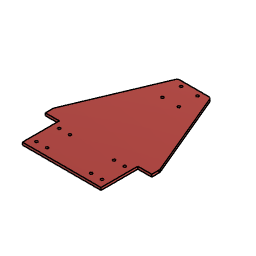
Chassis v45 (Autodesk Fusion 360 design; units mm, degrees)
Autodesk Fusion 360 part; units mm, degrees
sketch "Main" plane through (0, 0, 0) normal (0, 0, 1) x (1, 0, 0)
  line L0 (0, 55) -> (45, 162)
  line L1 (45, 162) -> (85, 162)
  line L2 (85, 162) -> (130, 55)
  line L3 (113, 0) -> (17, 0)
  line L4 (65, 0) -> (65, 162) construction
  line L5 (0, 55) -> (0, 45)
  line L6 (0, 45) -> (17, 45)
  line L7 (17, 45) -> (17, 0)
  line L8 (130, 55) -> (130, 45)
  line L9 (130, 45) -> (113, 45)
  line L10 (113, 45) -> (113, 0)
  dimension "d2" = 162
  dimension "d6" = 55
  dimension "d9" = 40
  dimension "d45" = 130
  dimension "d47" = 17
  dimension "d48" = 17
  dimension "d49" = 10
  dimension "d50" = 10
  constraint horizontal L0.start L2.end
  constraint midpoint L3 L4.start
  constraint perpendicular L3 L4
  constraint midpoint L1 L4.end
  constraint vertical L5
  constraint perpendicular L5 L6
  constraint coincident L3 L7.end
  constraint perpendicular L3 L7
  constraint vertical L8
  constraint perpendicular L8 L9
  constraint coincident L3 L10.end
  constraint perpendicular L3 L10
  constraint horizontal L3
  constraint coincident L3.start L10.end
  constraint vertical origin L5.end
  constraint coincident L3.end L7.end
  constraint horizontal origin L3.end
  measures "d2" distance of L1 L3
  measures "d6" distance of origin L0.start
  measures "d9" distance of L0.end L1.end
  measures "d45" distance of L5 L8
  measures "d47" distance of L5.end L6.end
  measures "d48" distance of L8.end L9.end
  measures "d49" distance of L2.end L8.end
  measures "d50" distance of L0.start L5.end
extrude "Extrude1" add sketch "Main" along normal blind 3
sketch "Head Tube Holes" plane through (0, 0, 3) normal (0, 0, 1) x (-1, 0, 0)
  line L0 (-17, 0) -> (-113, 0)
  line L1 (-130, -55) -> (-85, -162)
  line L2 (-85, -162) -> (-45, -162)
  line L3 (-45, -162) -> (0, -55)
  circle A0 centre (-55, -156) radius 1.55
  line L4 (-65, -162) -> (-65, 0) construction
  circle A1 centre (-75, -156) radius 1.55
  circle A2 centre (-55, -133) radius 1.55
  circle A3 centre (-75, -133) radius 1.55
  line L5 (0, -55) -> (0, -45)
  line L6 (0, -45) -> (-17, -45)
  line L7 (-17, -45) -> (-17, 0)
  line L8 (-113, 0) -> (-113, -45)
  line L9 (-113, -45) -> (-130, -45)
  line L10 (-130, -45) -> (-130, -55)
  dimension "d19" = 3.1
  dimension "d20" = 6
  dimension "d21" = 10
  dimension "d24" = -20
  dimension "d25" = 23
  constraint midpoint L2 L4.start
  constraint midpoint L0 L4.end
  measures "d19" diameter of A0
  measures "d20" distance of L2 A0.centre
  measures "d21" distance of A0.centre L4
extrude "Extrude2" cut sketch "Head Tube Holes" against normal up to surface (3 mm away) contours A0 | A1 | A2 | A3
sketch "Motor Box Holes" plane through (0, 0, 3) normal (0, 0, 1) x (-1, 0, 0)
  circle A0 centre (-75, -156) radius 1.55
  circle A1 centre (-55, -156) radius 1.55
  circle A2 centre (-75, -133) radius 1.55
  circle A3 centre (-55, -133) radius 1.55
  line L0 (-17, 0) -> (-113, 0)
  line L1 (-17, -37) -> (-113, -37) construction
  circle A4 centre (-25, -37) radius 1.55
  circle A5 centre (-38.1, -37) radius 1.55
  circle A6 centre (-25, -9.1) radius 1.55
  circle A7 centre (-38.1, -9.1) radius 1.55
  circle A8 centre (-105, -37) radius 1.55
  circle A9 centre (-91.9, -37) radius 1.55
  circle A10 centre (-105, -9.1) radius 1.55
  circle A11 centre (-91.9, -9.1) radius 1.55
  line L2 (-17, -45) -> (-17, 0)
  line L3 (-113, 0) -> (-113, -45)
  dimension "d30" = 3.1
  dimension "d32" = 37
  dimension "d35" = -13.1
  dimension "d36" = 27.9
  dimension "d37" = 3.1
  dimension "d40" = 13.1
  dimension "d41" = 27.9
  dimension "d53" = 8
  dimension "d54" = 8
  constraint coincident L1 A4.centre
  constraint coincident L1 A8.centre
  constraint coincident L1.end L3
  constraint coincident L1.start L2
  measures "d30" diameter of A4
  measures "d32" distance of L0 L1
  measures "d37" diameter of A8
  measures "d53" distance of A4.centre L2
  measures "d54" distance of A8.centre L3
extrude "Extrude3" cut sketch "Motor Box Holes" against normal through all contours A4 | A5 | A6 | A7 | A8 | A9 | A10 | A11
fillet "Fillet5" radius 3 2 edges at (45, 162, 1.5) (85, 162, 1.5)
fillet "Fillet6" radius 6 2 edges at (0, 55, 1.5) (130, 55, 1.5)
